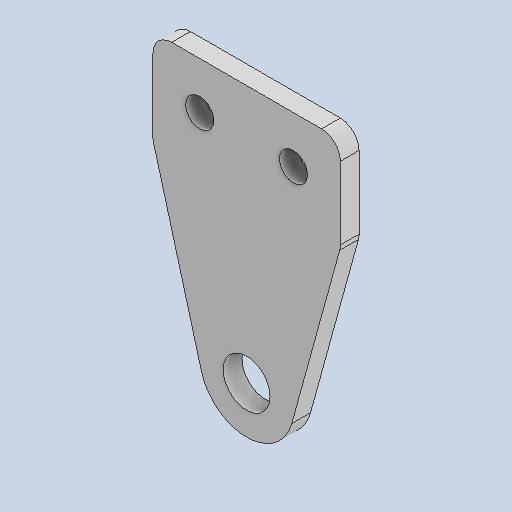
# Autodesk Inventor part: ballhand-v2-Plate-H-Air-F
Saved by Autodesk Inventor 2024 (Build 280153000, 153)
## iProperties
Created: 2024-03-17
Part Number: ballhand-v2-Plate-H-Air-F
Material: 一般
Document SubType Name: Modeling
Designer: haruy
Density: 1 g/cm^3
Appearance: 既定
Author: haruy
Autodesk Inventor part; units mm, degrees
ref_plane "YZ Plane" through (0, 0, 0) normal (1, 0, 0) x (0, 1, 0)
ref_plane "XZ Plane" through (0, 0, 0) normal (0, 1, 0) x (-1, 0, 0)
ref_plane "XY Plane" through (0, 0, 0) normal (0, 0, 1) x (1, 0, 0)
derived "ballhand-v2-Sketch-Base.ipt"
sketch "横から" plane through (0, 0, 0) normal (0, 0, 1) x (1, 0, 0)
  circle A0 centre (0, 0) radius 95
  line L0 (-321.6558, -95) -> (545.18, -95)
  line L1 (95, 81) -> (293, 81)
  line L2 (293, 81) -> (293, 61)
  line L3 (293, 61) -> (95, 61)
  line L4 (95, 61) -> (95, 81)
  line L5 (-52.5, 46.5) -> (145, 46.5)
  line L6 (145, 46.5) -> (145, 36.5)
  line L7 (145, 36.5) -> (-52.5, 36.5)
  line L8 (-52.5, 36.5) -> (-52.5, 46.5)
  line L9 (-52.5, -36.5) -> (145, -36.5)
  line L10 (145, -36.5) -> (145, -46.5)
  line L11 (145, -46.5) -> (-52.5, -46.5)
  line L12 (-52.5, -46.5) -> (-52.5, -36.5)
  line L13 (-50.5, 46.5) -> (-44.5, 46.5)
  line L14 (-44.5, 46.5) -> (-44.5, -46.5)
  line L15 (-44.5, -46.5) -> (-50.5, -46.5)
  line L16 (-50.5, -46.5) -> (-50.5, 46.5)
  line L17 (95, 5) -> (115, 5)
  line L18 (115, 5) -> (115, -5)
  line L19 (115, -5) -> (95, -5)
  line L20 (95, -5) -> (95, 5)
  line L21 (115, 4.5) -> (117.2, 4.5)
  line L22 (117.2, 4.5) -> (117.2, -4.5)
  line L23 (117.2, -4.5) -> (115, -4.5)
  line L24 (115, -4.5) -> (115, 4.5)
  line L25 (117.2, 10) -> (125, 10)
  line L26 (125, 10) -> (125, -10)
  line L27 (125, -10) -> (117.2, -10)
  line L28 (117.2, -10) -> (117.2, 10)
  line L29 (125, 46.5) -> (135, 46.5)
  line L30 (135, 46.5) -> (135, -46.5)
  line L31 (135, -46.5) -> (125, -46.5)
  line L32 (125, -46.5) -> (125, 46.5)
  line L33 (135, 36.5) -> (145, 36.5)
  line L34 (145, 36.5) -> (145, 26.5)
  line L35 (145, 26.5) -> (135, 26.5)
  line L36 (135, 26.5) -> (135, 36.5)
  line L37 (135, -36.5) -> (145, -36.5)
  line L38 (145, -36.5) -> (145, -26.5)
  line L39 (145, -26.5) -> (135, -26.5)
  line L40 (135, -26.5) -> (135, -36.5)
  line L41 (95, 33) -> (115, 33)
  line L42 (115, 33) -> (115, 43)
  line L43 (115, 43) -> (95, 43)
  line L44 (95, 43) -> (95, 33)
  line L45 (0, 0) -> (115, 0)
  line L46 (95, -33) -> (115, -33)
  line L47 (115, -43) -> (95, -43)
  line L48 (95, -43) -> (95, -33)
  line L49 (115, -33) -> (115, -43)
  line L50 (115, 81) -> (125, 81)
  line L51 (125, 81) -> (125, -43)
  line L52 (125, -43) -> (115, -43)
  line L53 (115, -43) -> (115, 81)
  circle A1 centre (105, 19) radius 2.5
  circle A2 centre (100, 41.5) radius 1.5
  circle A3 centre (110, 41.5) radius 1.5
  circle A4 centre (105, 19) radius 5
  line L54 (95, 46.5) -> (95, 36.5)
  line L55 (115, 46.5) -> (115, 36.5)
  line L56 (95, 36.5) -> (100.1791, 17.6738)
  line L57 (115, 36.5) -> (109.8209, 17.6738)
  point P0 (95, 36.5)
  point P1 (115, 46.5)
  dimension "d1" = 3
  dimension "d2" = 3
  dimension "d3" = 10
  dimension "d4" = 5
  dimension "d5" = 5
  dimension "d6" = 5
  dimension "d7" = 10
  dimension "d8" = 5
  dimension "d9" = 5
  measures "d1" diameter of A2
  measures "d2" diameter of A3
  measures "d3" distance of A2.centre A3.centre
  measures "d4" horizontal distance of A1.centre A3.centre
  measures "d5" distance from line of L7 A2.centre
  measures "d6" distance from line of A3.centre L7
  measures "d7" diameter of A4
  measures "d8" distance from line of A3.centre L55
  measures "d9" distance from line of L54 A2.centre
extrude "押し出し1" add sketch "横から" along normal blind 2 contours L44 L43 L42 L7 | L7 L57 L41 L56 | L5 L53 L43 L54 | L41 L57 A4 L56 | A4
fillet "フィレット1" radius 2 4 edges at (115, 46.5, 1) (115, 36.5, 1) (95, 36.5, 1) (95, 46.5, 1)
